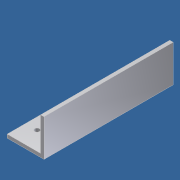
# Autodesk Inventor part: GE-12016-07
Saved by Autodesk Inventor 2012 (Build 160160000, 160)
## iProperties
Created: 2011-10-04
Part Number: GE-12016-07
Document SubType Name: Modeling
Designer: dfoster
Density: 1 g/cm^3
Description: Chute Bracket
Material: Default
Title: Chute Bracket
Author: dfoster
Autodesk Inventor part; units mm, degrees
ref_plane "YZ Plane" through (0, 0, 0) normal (1, 0, 0) x (0, 1, 0)
ref_plane "XZ Plane" through (0, 0, 0) normal (0, 1, 0) x (-1, 0, 0)
ref_plane "XY Plane" through (0, 0, 0) normal (0, 0, 1) x (1, 0, 0)
sketch "Sketch1" plane through (0, 0, 0) normal (0, 0, 1) x (1, 0, 0)
  line L0 (0, 50.8) -> (0, 0)
  line L1 (0, 0) -> (-50.8, 0)
  line L2 (-50.8, 0) -> (-50.8, 4.7752)
  line L3 (-50.8, 4.7752) -> (-4.7752, 4.7752)
  line L4 (-4.7752, 4.7752) -> (-4.7752, 50.8)
  line L5 (-4.7752, 50.8) -> (0, 50.8)
  dimension "d0" = 50.8
  dimension "d1" = 4.7752
  constraints: 12 end point, 4 parallel, 3 perpendicular, 1 vertical
  measures "d0" distance of L0.start L0.end
  measures "d1" distance between parallel lines of L4 L0
extrude "Extrusion1" add sketch "Sketch1" along normal blind 177.8
hole "Hole1" at (-34.925, 4.7752, 25.4) direction (0, -1, 0) diameter 6.731 depth 25.4 tip angle 118
hole "Hole2" at (-34.925, 4.7752, 152.4) direction (0, -1, 0) diameter 6.731 depth 25.4 tip angle 118
body "Solid1"
